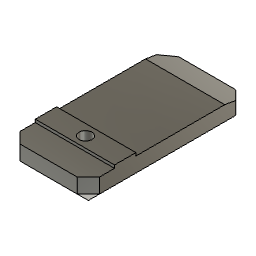
TopHat Aligners v3 (Autodesk Fusion 360 design; units mm, degrees)
Autodesk Fusion 360 part; units mm, degrees
note: some values were not read from the file. Set by a fixed rule: the direction of a hole.
sketch "Sketch1" plane through (0, 0, 0) normal (0, 0, 1) x (1, 0, 0)
  line L0 (0, 0) -> (21.5, 0)
  line L1 (21.5, 0) -> (21.5, 43)
  line L2 (21.5, 43) -> (0, 43)
  line L3 (0, 43) -> (0, 0)
  line L4 (0, 10) -> (21.5, 10) construction
  point P0 (10.75, 10)
  dimension "d1" = 21.5
  dimension "d2" = 43
  dimension "d3" = 10
  constraint horizontal L0
  constraint vertical L1
  constraint horizontal L2
  constraint vertical L3
  constraint coincident L0.start L3.end
  constraint coincident L3 L4.start
  constraint coincident L1 L4.end
  constraint perpendicular L1 L4
  constraint midpoint L4 P0
  measures "d1" distance of L0.start L0.end
  measures "d2" distance of L0.start L2.end
  measures "d3" distance of L0 L4
extrude "Extrude1" add sketch "Sketch1" along normal blind 7
sketch "Sketch3" plane through (0, 0, 7) normal (0, 0, 1) x (-1, 0, 0)
  line L0 (0, -43) -> (0, 0)
  line L1 (0, 0) -> (-21.5, 0)
  line L2 (-21.5, 0) -> (-21.5, -43)
  line L3 (-21.5, -43) -> (0, -43)
  line L4 (0, -10) -> (-21.5, -10)
  line L5 (0, -7.1) -> (-21.5, -7.1)
  line L6 (-21.5, -12.9) -> (0, -12.9)
  circle A0 centre (-10.75, -10) radius 1.75
  dimension "d12" = 2.9
  dimension "d13" = 2.9
  constraint coincident L0 L5.start
  constraint coincident L2 L5.end
  constraint perpendicular L2 L5
  constraint coincident L2 L6.start
  constraint coincident L0 L6.end
  constraint perpendicular L0 L6
  measures "d12" distance of L4 L5
  measures "d13" distance of L4 L6
extrude "Extrude2" add sketch "Sketch3" along normal blind 0.8 contours L0 L2 L4 L6 A0 | L0 L2 L4 L5 A0 | L4 A0 | L4 A0
sketch "Sketch2" plane through (0, 0, 0) normal (0, 0, 1) x (1, 0, 0)
hole "Hole1" at (10.75, 10, 0) direction (0, 0, 1) diameter 3.5 end through all counterbore diameter 6 counterbore depth 3
sketch "Sketch4" plane through (0, 0, 3) normal (0, 0, -1) x (1, 0, 0)
  circle A0 centre (10.75, -10) radius 3
  circle A1 centre (10.75, -10) radius 1.75
  line L0 (12.5, -13.6301) -> (12.5, -6.1711)
  line L1 (14.0891, -11.75) -> (6.0061, -11.75)
  line L2 (7.4109, -8.25) -> (15.4939, -8.25)
  line L3 (9, -6.3699) -> (9, -13.8289)
  constraint vertical L0
  constraint tangent A1 L0
  constraint horizontal L1
  constraint tangent A1 L1
  constraint tangent A1 L2
  constraint tangent A1 L3
extrude "Extrude3" add sketch "Sketch4" along normal blind 0.2 contours A0 L0 L1 L2 | A0 L0 L2 | A0 L0 L1 | A0 L2 L3 | A0 L1 L3 | A0 L1 L2 L3
extrude "Extrude4" cut sketch "Sketch4" against normal blind 0.2 contours A1 L0 L2 | A1 L0 L1 | A1 L2 L3 | A1 L1 L3
chamfer "Chamfer1" distance 3 angle 45 8 edges at (21.5, 0, 3.5) (10.75, 0, 0) (0, 21.5, 0) (10.75, 43, 0) (21.5, 21.5, 0) (0, 0, 3.5) (0, 43, 3.5) (21.5, 43, 3.5)
chamfer "Chamfer2" distance 6 distance2 1 1 edges at (10.75, 43, 7) measured on face at (7.1667, 30.9667, 7)
equation "d1 = ( 43 / 2 ) * 1 mm"
equation "d12 = SlotWidth / 2"
equation "d13 = SlotWidth / 2"
equation "SlotWidth = 5.8 mm"
